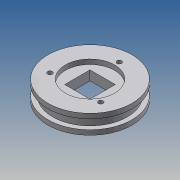
# Autodesk Inventor part: polea pequeña
Saved by Autodesk Inventor 2017 (Build 210142000, 142)
## iProperties
Part Number: polea pequeña
Material: Genérico
Document SubType Name: Modeling
Designer: FABLAB
Density: 1 g/cm^3
Appearance: Blanco
Description: Acrílico corte laser CNC
Author: FABLAB
Autodesk Inventor part; units mm, degrees
ref_plane "YZ Plane" through (0, 0, 0) normal (1, 0, 0) x (0, 1, 0)
ref_plane "XZ Plane" through (0, 0, 0) normal (0, 1, 0) x (-1, 0, 0)
ref_plane "XY Plane" through (0, 0, 0) normal (0, 0, 1) x (1, 0, 0)
sketch "Boceto1" plane through (0, 0, 0) normal (0, 0, 1) x (1, 0, 0)
  line L0 (8, -8) -> (-8, -8) projected
  line L1 (-8, -8) -> (-8, 8) projected
  line L2 (-8, 8) -> (8, 8) projected
  line L3 (8, 8) -> (8, -8) projected
  circle A0 centre (0, 0) radius 15 construction
  circle A1 centre (0, 0) radius 23.5
  circle A2 centre (0, 0) radius 18.5 construction
  circle A3 centre (0, 18.5) radius 1.5
  circle A4 centre (-16.0215, -9.25) radius 1.5
  circle A5 centre (16.0215, -9.25) radius 1.5
  dimension "d0" = 47
  dimension "d3" = 3
  dimension "d4" = 5
  dimension "d7" = 360
  constraints: 4 centre point, 2 coincident, 2 vertical alignment, 9 other
  measures "d0" diameter of A1
  measures "d3" diameter of A3
extrude "Extrusión1" add sketch "Boceto1" along normal blind 6
sketch "Boceto2" plane through (0, 0, 6) normal (0, 0, 1) x (1, 0, 0)
  circle A0 centre (0, 0) radius 26.5
  circle A1 centre (0, 0) radius 15.5
  circle A2 centre (0, 0) radius 23.5 construction
  circle A3 centre (0, 18.5) radius 1.5 projected
  circle A4 centre (16.0215, -9.25) radius 1.5 projected
  circle A5 centre (-16.0215, -9.25) radius 1.5 projected
  dimension "d9" = 31
  dimension "d10" = 3
  constraints: 2 centre point, 2 coincident
  measures "d9" diameter of A1
  measures "d10" radial gap between concentric circles of A0 A2
extrude "Extrusión2" add sketch "Boceto2" along normal blind 3 separate body
pattern_linear "Patrón rectangular1" count 2 spacing 9 along (0, 0, -1) bodies 2
